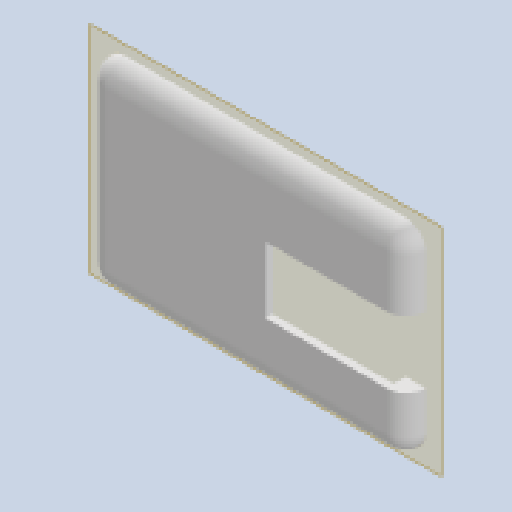
# Autodesk Inventor part: голова потолок
Saved by Autodesk Inventor 2024.2 (Build 282272000, 272)
## iProperties
Created: 2025-10-19
Part Number: голова потолок
Material: Типовые
Document SubType Name: Modeling
Designer: katya_notebook
Density: 1 g/cm^3
Appearance: По умолчанию
Author: katya_notebook
Autodesk Inventor part; units mm, degrees
ref_plane "YZ Plane" through (0, 0, 0) normal (1, 0, 0) x (0, 1, 0)
ref_plane "XZ Plane" through (0, 0, 0) normal (0, 1, 0) x (-1, 0, 0)
ref_plane "XY Plane" through (0, 0, 0) normal (0, 0, 1) x (1, 0, 0)
ref_plane "РабПлоскость1" through (0, 0, 0) normal (0, 0, 1) x (1, 0, 0)
sketch "Эскиз1" plane through (0, 0, 0) normal (0, 0, 1) x (1, 0, 0)
  line L0 (65, -32) -> (65, 32) projected
  line L1 (57, 40) -> (-57, 40) projected
  line L2 (-57, -40) -> (57, -40) projected
  line L3 (-65, 32) -> (-65, -32) projected
  line L4 (57, 40) -> (-57, 40)
  line L5 (-65, 32) -> (-65, -32)
  line L6 (-57, -40) -> (57, -40)
  line L7 (65, -32) -> (65, 32)
  arc A0 (65, 32) -> (57, 40) centre (57, 32) ccw
  arc A1 (-57, 40) -> (-65, 32) centre (-57, 32) ccw
  arc A2 (-65, -32) -> (-57, -40) centre (-57, -32) ccw
  arc A3 (57, -40) -> (65, -32) centre (57, -32) ccw
  point P0 (0, 0)
  constraints: 8 end point, 8 point on circle, 8 tangent, 4 centre point, 2 collinear, 1 horizontal, 1 perpendicular
extrude "Выдавливание1" add sketch "Эскиз1" along normal blind 8
fillet "Сопряжение1" radius 8 8 edges at (-62.6569, 37.6569, 8) (-65, 0, 8) (-62.6569, -37.6569, 8) (0, -40, 8) (62.6569, -37.6569, 8) (65, 0, 8) (62.6569, 37.6569, 8) (0, 40, 8)
sketch "Эскиз2" plane through (0, 0, 0) normal (0, 0, -1) x (-1, 0, 0)
  line L0 (57, 32) -> (-57, 32) projected
  line L1 (57, -32) -> (57, 32) projected
  line L2 (-57, -32) -> (57, -32) projected
  line L3 (-57, 32) -> (-57, -32) projected
  line L4 (-57, 32) -> (57, 32)
  line L5 (57, 32) -> (57, -32)
  line L6 (57, -32) -> (-57, -32)
  line L7 (-57, -32) -> (-57, 32)
  line L8 (-57, 32) -> (57, -32) construction
  line L9 (57, 32) -> (-57, -32) construction
  point P0 (0, 0)
  constraints: 12 end point, 2 midpoint, 2 parallel, 1 horizontal, 1 perpendicular
extrude "Выдавливание2" cut sketch "Эскиз2" against normal blind 5
sketch "Эскиз3" plane through (0, 0, 8) normal (0, 0, 1) x (1, 0, 0)
  line L0 (17.9625, 7.5) -> (17.9625, -12.5) projected
  line L1 (15.6638, -12.5) -> (138.4378, -12.5) projected
  line L2 (15.6638, 7.5) -> (138.4378, 7.5) projected
  line L3 (-15.6638, -12.5) -> (-138.4378, -12.5) projected
  line L4 (-15.6638, 7.5) -> (-138.4378, 7.5) projected
  line L5 (-15.6638, -12.5) -> (-15.6638, 7.5) projected
  line L6 (-17.9625, 7.5) -> (-17.9625, -12.5) projected
  line L7 (15.6638, 7.5) -> (15.6638, -12.5) projected
  line L8 (65, -32) -> (65, 32) projected
  line L9 (65, -12.5) -> (15.6638, -12.5)
  line L10 (15.6638, -12.5) -> (15.6638, 7.5)
  line L11 (40.3319, -12.5) -> (40.3319, 7.5)
  line L12 (15.6638, -2.5) -> (65, -2.5)
  line L13 (0, -39.4701) -> (0, 32)
  line L14 (57, 32) -> (-57, 32) projected
  line L15 (-40.3319, -12.5) -> (-40.3319, 7.5)
  line L16 (-15.6638, -2.5) -> (-65, -2.5)
  line L17 (7.8319, 11) -> (72.8319, 11)
  line L18 (72.8319, 11) -> (72.8319, -16)
  line L19 (72.8319, -16) -> (7.8319, -16)
  line L20 (7.8319, -16) -> (7.8319, 11)
  line L21 (7.8319, 11) -> (72.8319, -16) construction
  line L22 (72.8319, 11) -> (7.8319, -16) construction
  line L23 (-72.8319, 11) -> (-7.8319, 11)
  line L24 (-7.8319, 11) -> (-7.8319, -16)
  line L25 (-7.8319, -16) -> (-72.8319, -16)
  line L26 (-72.8319, -16) -> (-72.8319, 11)
  line L27 (-72.8319, 11) -> (-7.8319, -16) construction
  line L28 (-7.8319, 11) -> (-72.8319, -16) construction
  point P0 (0, 0)
  point P1 (40.3319, -2.5)
  point P2 (-40.3319, -2.5)
  dimension "d5" = 65
  dimension "d6" = 27
  dimension "d7" = 65
  dimension "d8" = 27
  constraints: 38 end point, 9 midpoint, 4 parallel, 4 perpendicular, 4 point on line, 4 symmetric about line, 2 collinear, 2 horizontal
  measures "d5" distance of L18.end L19.end
  measures "d6" distance of L19.end L17.start
  measures "d7" distance of L24.end L25.end
  measures "d8" distance of L23.end L24.end
extrude "Выдавливание3" cut sketch "Эскиз3" against normal blind 10
